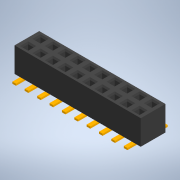
# Autodesk Inventor part: SMT10x2pin
Saved by Autodesk Inventor 2022 (Build 260153000, 153)
## iProperties
Created: 2024-12-15
Part Number: SMT10x2pin
Material: Типовые
Document SubType Name: Modeling
Designer: Andrey
Density: 1 g/cm^3
Appearance: По умолчанию
Author: Andrey
Autodesk Inventor part; units mm, degrees
ref_plane "YZ Plane" through (0, 0, 0) normal (1, 0, 0) x (0, 1, 0)
ref_plane "XZ Plane" through (0, 0, 0) normal (0, 1, 0) x (-1, 0, 0)
ref_plane "XY Plane" through (0, 0, 0) normal (0, 0, 1) x (1, 0, 0)
sketch "Эскиз1" plane through (0, 0, 0) normal (0, 1, 0) x (-1, 0, 0)
  line L0 (-10.2, 2) -> (10.2, 2)
  line L1 (10.2, 2) -> (10.2, -2)
  line L2 (10.2, -2) -> (-10.2, -2)
  line L3 (-10.2, -2) -> (-10.2, 2)
  line L4 (-10.2, 2) -> (10.2, -2) construction
  line L5 (10.2, 2) -> (-10.2, -2) construction
  line L6 (-9, 1) -> (9, 1)
  line L7 (9, 1) -> (9, -1)
  line L8 (9, -1) -> (-9, -1)
  line L9 (-9, -1) -> (-9, 1)
  line L10 (-9, 1) -> (9, -1) construction
  line L11 (9, 1) -> (-9, -1) construction
  line L12 (9.45, 1.45) -> (8.55, 1.45)
  line L13 (8.55, 1.45) -> (8.55, 0.55)
  line L14 (8.55, 0.55) -> (9.45, 0.55)
  line L15 (9.45, 0.55) -> (9.45, 1.45)
  line L16 (9.45, 1.45) -> (8.55, 0.55) construction
  line L17 (8.55, 1.45) -> (9.45, 0.55) construction
  line L18 (9, 1) -> (7, 1)
  line L19 (7, 1) -> (5, 1)
  line L20 (5, 1) -> (3, 1)
  line L21 (3, 1) -> (1, 1)
  line L22 (1, 1) -> (-1, 1)
  line L23 (-1, 1) -> (-3, 1)
  line L24 (-3, 1) -> (-5, 1)
  line L25 (-5, 1) -> (-7, 1)
  line L26 (9, -1) -> (7, -1)
  line L27 (7, -1) -> (5, -1)
  line L28 (5, -1) -> (3, -1)
  line L29 (3, -1) -> (1, -1)
  line L30 (1, -1) -> (-1, -1)
  line L31 (-1, -1) -> (-3, -1)
  line L32 (-3, -1) -> (-5, -1)
  line L33 (-5, -1) -> (-7, -1)
  line L34 (7.45, 1.45) -> (6.55, 1.45)
  line L35 (6.55, 1.45) -> (6.55, 0.55)
  line L36 (6.55, 0.55) -> (7.45, 0.55)
  line L37 (7.45, 0.55) -> (7.45, 1.45)
  line L38 (7.45, 1.45) -> (6.55, 0.55) construction
  line L39 (6.55, 1.45) -> (7.45, 0.55) construction
  line L40 (5.45, 1.45) -> (4.55, 1.45)
  line L41 (4.55, 1.45) -> (4.55, 0.55)
  line L42 (4.55, 0.55) -> (5.45, 0.55)
  line L43 (5.45, 0.55) -> (5.45, 1.45)
  line L44 (5.45, 1.45) -> (4.55, 0.55) construction
  line L45 (4.55, 1.45) -> (5.45, 0.55) construction
  line L46 (3.45, 1.45) -> (2.55, 1.45)
  line L47 (2.55, 1.45) -> (2.55, 0.55)
  line L48 (2.55, 0.55) -> (3.45, 0.55)
  line L49 (3.45, 0.55) -> (3.45, 1.45)
  line L50 (3.45, 1.45) -> (2.55, 0.55) construction
  line L51 (2.55, 1.45) -> (3.45, 0.55) construction
  line L52 (1.45, 1.45) -> (0.55, 1.45)
  line L53 (0.55, 1.45) -> (0.55, 0.55)
  line L54 (0.55, 0.55) -> (1.45, 0.55)
  line L55 (1.45, 0.55) -> (1.45, 1.45)
  line L56 (1.45, 1.45) -> (0.55, 0.55) construction
  line L57 (0.55, 1.45) -> (1.45, 0.55) construction
  line L58 (-0.55, 1.45) -> (-1.45, 1.45)
  line L59 (-1.45, 1.45) -> (-1.45, 0.55)
  line L60 (-1.45, 0.55) -> (-0.55, 0.55)
  line L61 (-0.55, 0.55) -> (-0.55, 1.45)
  line L62 (-0.55, 1.45) -> (-1.45, 0.55) construction
  line L63 (-1.45, 1.45) -> (-0.55, 0.55) construction
  line L64 (-2.55, 1.45) -> (-3.45, 1.45)
  line L65 (-3.45, 1.45) -> (-3.45, 0.55)
  line L66 (-3.45, 0.55) -> (-2.55, 0.55)
  line L67 (-2.55, 0.55) -> (-2.55, 1.45)
  line L68 (-2.55, 1.45) -> (-3.45, 0.55) construction
  line L69 (-3.45, 1.45) -> (-2.55, 0.55) construction
  line L70 (-4.55, 1.45) -> (-5.45, 1.45)
  line L71 (-5.45, 1.45) -> (-5.45, 0.55)
  line L72 (-5.45, 0.55) -> (-4.55, 0.55)
  line L73 (-4.55, 0.55) -> (-4.55, 1.45)
  line L74 (-4.55, 1.45) -> (-5.45, 0.55) construction
  line L75 (-5.45, 1.45) -> (-4.55, 0.55) construction
  line L76 (-6.55, 1.45) -> (-7.45, 1.45)
  line L77 (-7.45, 1.45) -> (-7.45, 0.55)
  line L78 (-7.45, 0.55) -> (-6.55, 0.55)
  line L79 (-6.55, 0.55) -> (-6.55, 1.45)
  line L80 (-6.55, 1.45) -> (-7.45, 0.55) construction
  line L81 (-7.45, 1.45) -> (-6.55, 0.55) construction
  line L82 (-8.55, 1.45) -> (-9.45, 1.45)
  line L83 (-9.45, 1.45) -> (-9.45, 0.55)
  line L84 (-9.45, 0.55) -> (-8.55, 0.55)
  line L85 (-8.55, 0.55) -> (-8.55, 1.45)
  line L86 (-8.55, 1.45) -> (-9.45, 0.55) construction
  line L87 (-9.45, 1.45) -> (-8.55, 0.55) construction
  line L88 (-8.55, -0.55) -> (-9.45, -0.55)
  line L89 (-9.45, -0.55) -> (-9.45, -1.45)
  line L90 (-9.45, -1.45) -> (-8.55, -1.45)
  line L91 (-8.55, -1.45) -> (-8.55, -0.55)
  line L92 (-8.55, -0.55) -> (-9.45, -1.45) construction
  line L93 (-9.45, -0.55) -> (-8.55, -1.45) construction
  line L94 (-6.55, -0.55) -> (-7.45, -0.55)
  line L95 (-7.45, -0.55) -> (-7.45, -1.45)
  line L96 (-7.45, -1.45) -> (-6.55, -1.45)
  line L97 (-6.55, -1.45) -> (-6.55, -0.55)
  line L98 (-6.55, -0.55) -> (-7.45, -1.45) construction
  line L99 (-7.45, -0.55) -> (-6.55, -1.45) construction
  line L100 (-4.55, -0.55) -> (-5.45, -0.55)
  line L101 (-5.45, -0.55) -> (-5.45, -1.45)
  line L102 (-5.45, -1.45) -> (-4.55, -1.45)
  line L103 (-4.55, -1.45) -> (-4.55, -0.55)
  line L104 (-4.55, -0.55) -> (-5.45, -1.45) construction
  line L105 (-5.45, -0.55) -> (-4.55, -1.45) construction
  line L106 (-0.5574, -0.5122) -> (-1.4574, -0.5122)
  line L107 (-1.4574, -0.5122) -> (-1.4574, -1.4122)
  line L108 (-1.4574, -1.4122) -> (-0.5574, -1.4122)
  line L109 (-0.5574, -1.4122) -> (-0.5574, -0.5122)
  line L110 (-0.5574, -0.5122) -> (-1.4574, -1.4122) construction
  line L111 (-1.4574, -0.5122) -> (-0.5574, -1.4122) construction
  line L112 (-2.55, -0.55) -> (-3.45, -0.55)
  line L113 (-3.45, -0.55) -> (-3.45, -1.45)
  line L114 (-3.45, -1.45) -> (-2.55, -1.45)
  line L115 (-2.55, -1.45) -> (-2.55, -0.55)
  line L116 (-2.55, -0.55) -> (-3.45, -1.45) construction
  line L117 (-3.45, -0.55) -> (-2.55, -1.45) construction
  line L118 (9.45, -0.55) -> (8.55, -0.55)
  line L119 (8.55, -0.55) -> (8.55, -1.45)
  line L120 (8.55, -1.45) -> (9.45, -1.45)
  line L121 (9.45, -1.45) -> (9.45, -0.55)
  line L122 (9.45, -0.55) -> (8.55, -1.45) construction
  line L123 (8.55, -0.55) -> (9.45, -1.45) construction
  line L124 (9, -1) -> (7, -1)
  line L125 (7, -1) -> (5, -1)
  line L126 (5, -1) -> (3, -1)
  line L127 (3, -1) -> (1, -1)
  line L128 (7.45, -0.55) -> (6.55, -0.55)
  line L129 (6.55, -0.55) -> (6.55, -1.45)
  line L130 (6.55, -1.45) -> (7.45, -1.45)
  line L131 (7.45, -1.45) -> (7.45, -0.55)
  line L132 (7.45, -0.55) -> (6.55, -1.45) construction
  line L133 (6.55, -0.55) -> (7.45, -1.45) construction
  line L134 (5.45, -0.55) -> (4.55, -0.55)
  line L135 (4.55, -0.55) -> (4.55, -1.45)
  line L136 (4.55, -1.45) -> (5.45, -1.45)
  line L137 (5.45, -1.45) -> (5.45, -0.55)
  line L138 (5.45, -0.55) -> (4.55, -1.45) construction
  line L139 (4.55, -0.55) -> (5.45, -1.45) construction
  line L140 (3.45, -0.55) -> (2.55, -0.55)
  line L141 (2.55, -0.55) -> (2.55, -1.45)
  line L142 (2.55, -1.45) -> (3.45, -1.45)
  line L143 (3.45, -1.45) -> (3.45, -0.55)
  line L144 (3.45, -0.55) -> (2.55, -1.45) construction
  line L145 (2.55, -0.55) -> (3.45, -1.45) construction
  line L146 (1.45, -0.55) -> (0.55, -0.55)
  line L147 (0.55, -0.55) -> (0.55, -1.45)
  line L148 (0.55, -1.45) -> (1.45, -1.45)
  line L149 (1.45, -1.45) -> (1.45, -0.55)
  line L150 (1.45, -0.55) -> (0.55, -1.45) construction
  line L151 (0.55, -0.55) -> (1.45, -1.45) construction
  point P0 (0, 0)
  point P1 (3, 1)
  point P2 (-1, 1)
  point P3 (-5, 1)
  point P4 (-7, 1)
  point P5 (-7, -1)
  point P6 (-5, -1)
  point P7 (-1.0074, -0.9622)
  point P8 (-3, -1)
  point P9 (3, -1)
  dimension "d0" = 20.4
  dimension "d1" = 4
  dimension "d2" = 18
  dimension "d3" = 2
  dimension "d4" = 0.9
  dimension "d5" = 0.9
  dimension "d6" = 2
  dimension "d7" = 2
  dimension "d8" = 2
  dimension "d9" = 2
  dimension "d10" = 2
  dimension "d11" = 2
  dimension "d12" = 2
  dimension "d13" = 2
  dimension "d14" = 2
  dimension "d15" = 2
  dimension "d16" = 2
  dimension "d17" = 2
  dimension "d18" = 2
  dimension "d19" = 2
  dimension "d20" = 2
  dimension "d21" = 2
  dimension "d22" = 0.9
  dimension "d23" = 0.9
  dimension "d24" = 0.9
  dimension "d25" = 0.9
  dimension "d26" = 0.9
  dimension "d27" = 0.9
  dimension "d28" = 0.9
  dimension "d29" = 0.9
  dimension "d30" = 0.9
  dimension "d31" = 0.9
  dimension "d32" = 0.9
  dimension "d33" = 0.9
  dimension "d34" = 0.9
  dimension "d35" = 0.9
  dimension "d36" = 0.9
  dimension "d37" = 0.9
  dimension "d38" = 0.9
  dimension "d39" = 0.9
  dimension "d40" = 0.9
  dimension "d41" = 0.9
  dimension "d42" = 0.9
  dimension "d43" = 0.9
  dimension "d44" = 0.9
  dimension "d45" = 0.9
  dimension "d46" = 0.9
  dimension "d47" = 0.9
  dimension "d48" = 0.9
  dimension "d49" = 0.9
  dimension "d50" = 0.9
  dimension "d51" = 0.9
  dimension "d52" = 2
  dimension "d53" = 2
  dimension "d54" = 2
  dimension "d55" = 2
  dimension "d56" = 0.9
  dimension "d57" = 0.9
  dimension "d58" = 0.9
  dimension "d59" = 0.9
  dimension "d60" = 0.9
  dimension "d61" = 0.9
  dimension "d62" = 0.9
  dimension "d63" = 0.9
  constraints: 300 end point, 44 midpoint, 43 parallel, 21 horizontal, 21 perpendicular, 1 vertical, 22 other
  measures "d0" distance of L1.end L2.end
  measures "d1" distance of L0.end L1.end
  measures "d2" distance of L7.end L9.start
  measures "d3" distance of L7.start L7.end
  measures "d4" distance of L14.end L13.end
  measures "d5" distance of L13.end L12.end
  measures "d6" distance of L7.start L18.end
  measures "d7" distance of L18.end L19.end
  measures "d8" distance of L19.end L20.end
  measures "d9" distance of L20.end L21.end
  measures "d10" distance of L21.end L22.end
  measures "d11" distance of L22.end L23.end
  measures "d12" distance of L23.end L24.end
  measures "d13" distance of L24.end L25.end
  measures "d14" distance of L7.end L26.end
  measures "d15" distance of L26.end L27.end
  measures "d16" distance of L27.end L28.end
  measures "d17" distance of L28.end L29.end
  measures "d18" distance of L29.end L30.end
  measures "d19" distance of L30.end L31.end
  measures "d20" distance of L31.end L32.end
  measures "d21" distance of L32.end L33.end
  measures "d22" distance of L36.end L35.end
  measures "d23" distance of L35.end L34.end
  measures "d24" distance of L42.end L41.end
  measures "d25" distance of L41.end L40.end
  measures "d26" distance of L48.end L47.end
  measures "d27" distance of L47.end L46.end
  measures "d28" distance of L54.end L53.end
  measures "d29" distance of L53.end L52.end
  measures "d30" distance of L60.end L59.end
  measures "d31" distance of L59.end L58.end
  measures "d32" distance of L66.end L65.end
  measures "d33" distance of L65.end L64.end
  measures "d34" distance of L72.end L71.end
  measures "d35" distance of L71.end L70.end
  measures "d36" distance of L78.end L77.end
  measures "d37" distance of L77.end L76.end
  measures "d38" distance of L84.end L83.end
  measures "d39" distance of L83.end L82.end
  measures "d40" distance of L90.end L89.end
  measures "d41" distance of L89.end L88.end
  measures "d42" distance of L96.end L95.end
  measures "d43" distance of L95.end L94.end
  measures "d44" distance of L102.end L101.end
  measures "d45" distance of L101.end L100.end
  measures "d46" distance of L108.end L107.end
  measures "d47" distance of L107.end L106.end
  measures "d48" distance of L114.end L113.end
  measures "d49" distance of L113.end L112.end
  measures "d50" distance of L121.start L119.end
  measures "d51" distance of L119.end L118.end
  measures "d52" distance of L124.start L125.start
  measures "d53" distance of L125.start L125.end
  measures "d54" distance of L125.end L126.end
  measures "d55" distance of L126.end L127.end
  measures "d56" distance of L130.end L129.end
  measures "d57" distance of L129.end L129.start
  measures "d58" distance of L137.start L135.end
  measures "d59" distance of L135.end L135.start
  measures "d60" distance of L142.end L141.end
  measures "d61" distance of L141.end L141.start
  measures "d62" distance of L149.start L148.start
  measures "d63" distance of L148.start L147.start
extrude "Выдавливание1" add sketch "Эскиз1" along normal blind 4 contours L0 L1 L2 L3 | L6 L77 L78 L79 L71 L72 L73 L65 L66 L67 L59 L60 L61 L53 L54 L55 L47 L48 L49 L41 L42 L43 L35 L36 L37 L13 L14 L7 L118 L119 L8 L131 L128 L129 L137 L134 L135 L143 L140 L141 L149 L146 L147 L109 L106 L107 L115 L112 L113 L103 L100 L101 L97 L94 L95 L91 L88 L9 L84 L85
chamfer "Фаска1" distance 0.2 angle 45 80 edges at (4.55, 4, 1) (5.45, 4, 1) (5, 4, -0.55) (-8.55, 4, 1) (-9, 4, 1.45) (-9.45, 4, 1) (-9.45, 4, -1) (-9, 4, 0.55) (-9, 4, -0.55) (-1.45, 4, 1) (-2.55, 4, 1) (3.45, 4, -1) (2.55, 4, -1) (-3.45, 4, -1) (-2.55, 4, -1) (-3, 4, -0.55) (-3, 4, -1.45) (-3, 4, 1.45) (-3, 4, 0.55) (-3.45, 4, 1) (-4.55, 4, 1) (-5, 4, 1.45) (-7.45, 4, -1) (-7, 4, -1.45) (-6.55, 4, -1) (-7, 4, -0.55) (-5, 4, 0.55) (-6.55, 4, 1) (-7.45, 4, 1) (-7, 4, 0.55) (-5.45, 4, 1) (-7, 4, 1.45) (-8.55, 4, -1) (-9, 4, -1.45) (-5.45, 4, -1) (-5, 4, -1.45) (-4.55, 4, -1) (-5, 4, -0.55) (-1.45, 4, -1) (-0.55, 4, -1) (-1, 4, -1.45) (-1, 4, -0.55) (-1, 4, 0.55) (0.55, 4, 1) (-0.55, 4, 1) (1.45, 4, 1) (1, 4, 0.55) (1, 4, 1.45) (1.4574, 4, -0.9622) (0.5574, 4, -0.9622) (1.0074, 4, -1.4122) (1.0074, 4, -0.5122) (-1, 4, 1.45) (2.55, 4, 1) (3, 4, -0.55) (3, 4, 0.55) (3, 4, 1.45) (3.45, 4, 1) (5, 4, 0.55) (5, 4, 1.45) (5.45, 4, -1) (4.55, 4, -1) (5, 4, -1.45) (6.55, 4, -1) (7, 4, -1.45) (7.45, 4, -1) (7, 4, -0.55) (7.45, 4, 1) (7, 4, 1.45) (6.55, 4, 1) (7, 4, 0.55) (8.55, 4, -1) (9, 4, -1.45) (9.45, 4, -1) (9, 4, -0.55) (9, 4, 0.55) (9.45, 4, 1) (9, 4, 1.45) (8.55, 4, 1) (3, 4, -1.45)
sketch "Эскиз2" plane through (0, 0, 0) normal (0, -1, 0) x (1, 0, 0)
  line L0 (-9.45, 0.55) -> (-8.55, 0.55) projected
  line L1 (-9, 0.55) -> (-9, -0.55)
  line L2 (-8.55, -0.55) -> (-9.45, -0.55) projected
  line L3 (10.2, -2) -> (-10.2, -2) projected
  line L4 (10.2, 2) -> (10.2, -2) projected
  line L5 (-10.2, 2) -> (10.2, 2) projected
  line L6 (-10.2, -2) -> (-10.2, 2) projected
  line L7 (-8.55, 0.55) -> (-8.55, 1.45) projected
  line L8 (-9.45, 0.55) -> (-8.55, 0.55) projected
  line L9 (-9.45, 1.45) -> (-9.45, 0.55) projected
  line L10 (-8.55, 1.45) -> (-9.45, 1.45) projected
  line L11 (-8.55, -0.55) -> (-9.45, -0.55) projected
  line L12 (-8.55, -1.45) -> (-8.55, -0.55) projected
  line L13 (-9.45, -1.45) -> (-8.55, -1.45) projected
  line L14 (-9.45, -0.55) -> (-9.45, -1.45) projected
  line L15 (-7.45, -0.55) -> (-7.45, -1.45) projected
  line L16 (-6.55, -0.55) -> (-7.45, -0.55) projected
  line L17 (-6.55, -1.45) -> (-6.55, -0.55) projected
  line L18 (-7.45, -1.45) -> (-6.55, -1.45) projected
  line L19 (-5.45, -0.55) -> (-5.45, -1.45) projected
  line L20 (-4.55, -0.55) -> (-5.45, -0.55) projected
  line L21 (-4.55, -1.45) -> (-4.55, -0.55) projected
  line L22 (-5.45, -1.45) -> (-4.55, -1.45) projected
  line L23 (-3.45, -0.55) -> (-3.45, -1.45) projected
  line L24 (-2.55, -0.55) -> (-3.45, -0.55) projected
  line L25 (-2.55, -1.45) -> (-2.55, -0.55) projected
  line L26 (-3.45, -1.45) -> (-2.55, -1.45) projected
  line L27 (-1.45, -0.55) -> (-1.45, -1.45) projected
  line L28 (-0.55, -0.55) -> (-1.45, -0.55) projected
  line L29 (-0.55, -1.45) -> (-0.55, -0.55) projected
  line L30 (-1.45, -1.45) -> (-0.55, -1.45) projected
  line L31 (0.5574, -0.5122) -> (0.5574, -1.4122) projected
  line L32 (1.4574, -0.5122) -> (0.5574, -0.5122) projected
  line L33 (1.4574, -1.4122) -> (1.4574, -0.5122) projected
  line L34 (0.5574, -1.4122) -> (1.4574, -1.4122) projected
  line L35 (2.55, -0.55) -> (2.55, -1.45) projected
  line L36 (3.45, -0.55) -> (2.55, -0.55) projected
  line L37 (3.45, -1.45) -> (3.45, -0.55) projected
  line L38 (2.55, -1.45) -> (3.45, -1.45) projected
  line L39 (4.55, -0.55) -> (4.55, -1.45) projected
  line L40 (5.45, -0.55) -> (4.55, -0.55) projected
  line L41 (5.45, -1.45) -> (5.45, -0.55) projected
  line L42 (4.55, -1.45) -> (5.45, -1.45) projected
  line L43 (6.55, -0.55) -> (6.55, -1.45) projected
  line L44 (7.45, -0.55) -> (6.55, -0.55) projected
  line L45 (7.45, -1.45) -> (7.45, -0.55) projected
  line L46 (6.55, -1.45) -> (7.45, -1.45) projected
  line L47 (8.55, -0.55) -> (8.55, -1.45) projected
  line L48 (9.45, -0.55) -> (8.55, -0.55) projected
  line L49 (9.45, -1.45) -> (9.45, -0.55) projected
  line L50 (8.55, -1.45) -> (9.45, -1.45) projected
  line L51 (8.55, 0.55) -> (9.45, 0.55) projected
  line L52 (8.55, 1.45) -> (8.55, 0.55) projected
  line L53 (9.45, 1.45) -> (8.55, 1.45) projected
  line L54 (9.45, 0.55) -> (9.45, 1.45) projected
  line L55 (7.45, 0.55) -> (7.45, 1.45) projected
  line L56 (6.55, 0.55) -> (7.45, 0.55) projected
  line L57 (6.55, 1.45) -> (6.55, 0.55) projected
  line L58 (7.45, 1.45) -> (6.55, 1.45) projected
  line L59 (5.45, 0.55) -> (5.45, 1.45) projected
  line L60 (4.55, 0.55) -> (5.45, 0.55) projected
  line L61 (4.55, 1.45) -> (4.55, 0.55) projected
  line L62 (5.45, 1.45) -> (4.55, 1.45) projected
  line L63 (3.45, 0.55) -> (3.45, 1.45) projected
  line L64 (2.55, 0.55) -> (3.45, 0.55) projected
  line L65 (2.55, 1.45) -> (2.55, 0.55) projected
  line L66 (3.45, 1.45) -> (2.55, 1.45) projected
  line L67 (1.45, 0.55) -> (1.45, 1.45) projected
  line L68 (0.55, 0.55) -> (1.45, 0.55) projected
  line L69 (0.55, 1.45) -> (0.55, 0.55) projected
  line L70 (1.45, 1.45) -> (0.55, 1.45) projected
  line L71 (-0.55, 0.55) -> (-0.55, 1.45) projected
  line L72 (-1.45, 0.55) -> (-0.55, 0.55) projected
  line L73 (-1.45, 1.45) -> (-1.45, 0.55) projected
  line L74 (-0.55, 1.45) -> (-1.45, 1.45) projected
  line L75 (-2.55, 0.55) -> (-2.55, 1.45) projected
  line L76 (-3.45, 0.55) -> (-2.55, 0.55) projected
  line L77 (-3.45, 1.45) -> (-3.45, 0.55) projected
  line L78 (-2.55, 1.45) -> (-3.45, 1.45) projected
  line L79 (-4.55, 0.55) -> (-4.55, 1.45) projected
  line L80 (-5.45, 0.55) -> (-4.55, 0.55) projected
  line L81 (-5.45, 1.45) -> (-5.45, 0.55) projected
  line L82 (-4.55, 1.45) -> (-5.45, 1.45) projected
  line L83 (-7.45, 1.45) -> (-7.45, 0.55) projected
  line L84 (-6.55, 1.45) -> (-7.45, 1.45) projected
  line L85 (-6.55, 0.55) -> (-6.55, 1.45) projected
  line L86 (-7.45, 0.55) -> (-6.55, 0.55) projected
  line L87 (-9.3, -3.25) -> (-8.7, -3.25)
  line L88 (-8.7, -3.25) -> (-8.7, 3.25)
  line L89 (-8.7, 3.25) -> (-9.3, 3.25)
  line L90 (-9.3, 3.25) -> (-9.3, -3.25)
  line L91 (-9.3, -3.25) -> (-8.7, 3.25) construction
  line L92 (-8.7, -3.25) -> (-9.3, 3.25) construction
  line L93 (-7, 0.55) -> (-7, -0.55)
  line L94 (-7.3, -3.25) -> (-6.7, -3.25)
  line L95 (-6.7, -3.25) -> (-6.7, 3.25)
  line L96 (-6.7, 3.25) -> (-7.3, 3.25)
  line L97 (-7.3, 3.25) -> (-7.3, -3.25)
  line L98 (-7.3, -3.25) -> (-6.7, 3.25) construction
  line L99 (-6.7, -3.25) -> (-7.3, 3.25) construction
  line L100 (-5, 0.55) -> (-5, -0.55)
  line L101 (-5.3, -3.25) -> (-4.7, -3.25)
  line L102 (-4.7, -3.25) -> (-4.7, 3.25)
  line L103 (-4.7, 3.25) -> (-5.3, 3.25)
  line L104 (-5.3, 3.25) -> (-5.3, -3.25)
  line L105 (-5.3, -3.25) -> (-4.7, 3.25) construction
  line L106 (-4.7, -3.25) -> (-5.3, 3.25) construction
  line L107 (-3, 0.55) -> (-3, -0.55)
  line L108 (-3.3, -3.25) -> (-2.7, -3.25)
  line L109 (-2.7, -3.25) -> (-2.7, 3.25)
  line L110 (-2.7, 3.25) -> (-3.3, 3.25)
  line L111 (-3.3, 3.25) -> (-3.3, -3.25)
  line L112 (-3.3, -3.25) -> (-2.7, 3.25) construction
  line L113 (-2.7, -3.25) -> (-3.3, 3.25) construction
  line L114 (-1, 0.55) -> (-1, -0.55)
  line L115 (-1.3, -3.25) -> (-0.7, -3.25)
  line L116 (-0.7, -3.25) -> (-0.7, 3.25)
  line L117 (-0.7, 3.25) -> (-1.3, 3.25)
  line L118 (-1.3, 3.25) -> (-1.3, -3.25)
  line L119 (-1.3, -3.25) -> (-0.7, 3.25) construction
  line L120 (-0.7, -3.25) -> (-1.3, 3.25) construction
  line L121 (1, 0.55) -> (1, -0.55)
  line L122 (0.7, -3.25) -> (1.3, -3.25)
  line L123 (1.3, -3.25) -> (1.3, 3.25)
  line L124 (1.3, 3.25) -> (0.7, 3.25)
  line L125 (0.7, 3.25) -> (0.7, -3.25)
  line L126 (0.7, -3.25) -> (1.3, 3.25) construction
  line L127 (1.3, -3.25) -> (0.7, 3.25) construction
  line L128 (3, 0.55) -> (3, -0.55)
  line L129 (2.7, -3.25) -> (3.3, -3.25)
  line L130 (3.3, -3.25) -> (3.3, 3.25)
  line L131 (3.3, 3.25) -> (2.7, 3.25)
  line L132 (2.7, 3.25) -> (2.7, -3.25)
  line L133 (2.7, -3.25) -> (3.3, 3.25) construction
  line L134 (3.3, -3.25) -> (2.7, 3.25) construction
  line L135 (5, 0.55) -> (5, -0.55)
  line L136 (4.7, -3.25) -> (5.3, -3.25)
  line L137 (5.3, -3.25) -> (5.3, 3.25)
  line L138 (5.3, 3.25) -> (4.7, 3.25)
  line L139 (4.7, 3.25) -> (4.7, -3.25)
  line L140 (4.7, -3.25) -> (5.3, 3.25) construction
  line L141 (5.3, -3.25) -> (4.7, 3.25) construction
  line L142 (7, 0.55) -> (7, -0.55)
  line L143 (6.7, -3.25) -> (7.3, -3.25)
  line L144 (7.3, -3.25) -> (7.3, 3.25)
  line L145 (7.3, 3.25) -> (6.7, 3.25)
  line L146 (6.7, 3.25) -> (6.7, -3.25)
  line L147 (6.7, -3.25) -> (7.3, 3.25) construction
  line L148 (7.3, -3.25) -> (6.7, 3.25) construction
  line L149 (9, 0.55) -> (9, -0.55)
  line L150 (8.7, -3.25) -> (9.3, -3.25)
  line L151 (9.3, -3.25) -> (9.3, 3.25)
  line L152 (9.3, 3.25) -> (8.7, 3.25)
  line L153 (8.7, 3.25) -> (8.7, -3.25)
  line L154 (8.7, -3.25) -> (9.3, 3.25) construction
  line L155 (9.3, -3.25) -> (8.7, 3.25) construction
  point P0 (0, 0)
  point P1 (-9, 0)
  point P2 (-9.3, -1.45)
  point P3 (-8.7, -1.45)
  point P4 (-9.3, 1.45)
  point P5 (-8.7, 1.45)
  point P6 (-7, 0)
  point P7 (-5, 0)
  point P8 (-3, 0)
  point P9 (-1, 0)
  point P10 (1, 0)
  point P11 (3, 0)
  point P12 (5, 0)
  point P13 (7, 0)
  point P14 (9, 0)
  point P15 (6.7, 1.45)
  point P16 (7.3, 1.45)
  point P17 (8.7, 1.45)
  point P18 (9.3, 1.45)
  point P19 (4.7, 1.45)
  point P20 (5.3, 1.45)
  point P21 (2.7, 1.45)
  point P22 (3.3, 1.45)
  point P23 (0.7, 1.45)
  point P24 (1.3, 1.45)
  point P25 (-1.3, 1.45)
  point P26 (-0.7, 1.45)
  point P27 (-3.3, 1.45)
  point P28 (-2.7, 1.45)
  point P29 (7.3, -1.45)
  point P30 (6.7, -1.45)
  point P31 (9.3, -1.45)
  point P32 (8.7, -1.45)
  point P33 (5.3, -1.45)
  point P34 (4.7, -1.45)
  point P35 (3.3, -1.45)
  point P36 (2.7, -1.45)
  point P37 (1.3, -1.4122)
  point P38 (0.7, -1.4122)
  point P39 (-0.7, -1.45)
  point P40 (-1.3, -1.45)
  point P41 (-2.7, -1.45)
  point P42 (-3.3, -1.45)
  point P43 (-5.3, -1.45)
  point P44 (-4.7, -1.45)
  point P45 (-5.3, 1.45)
  point P46 (-4.7, 1.45)
  point P47 (-7.3, 1.45)
  point P48 (-6.7, 1.45)
  point P49 (-6.7, -1.45)
  point P50 (-7.3, -1.45)
  dimension "d69" = 0.6
  dimension "d70" = 6.5
  dimension "d91" = 0.6
  dimension "d92" = 6.5
  dimension "d93" = 0.6
  dimension "d94" = 6.5
  dimension "d95" = 0.6
  dimension "d96" = 6.5
  dimension "d97" = 0.6
  dimension "d98" = 6.5
  dimension "d99" = 0.6
  dimension "d100" = 6.5
  dimension "d101" = 0.6
  dimension "d102" = 6.5
  dimension "d103" = 0.6
  dimension "d104" = 6.5
  dimension "d105" = 0.6
  dimension "d106" = 6.5
  dimension "d107" = 0.6
  dimension "d108" = 6.5
  constraints: 140 end point, 32 midpoint, 20 parallel, 10 horizontal, 10 perpendicular
  measures "d69" distance between parallel lines of L88 L90
  measures "d70" distance of L89.end L87.start
  measures "d91" distance between parallel lines of L95 L97
  measures "d92" distance of L99.end L94.start
  measures "d93" distance between parallel lines of L102 L104
  measures "d94" distance of L106.end L101.start
  measures "d95" distance between parallel lines of L109 L111
  measures "d96" distance of L113.end L108.start
  measures "d97" distance between parallel lines of L116 L118
  measures "d98" distance of L120.end L115.start
  measures "d99" distance between parallel lines of L123 L125
  measures "d100" distance of L127.end L122.start
  measures "d101" distance between parallel lines of L130 L132
  measures "d102" distance of L134.end L129.start
  measures "d103" distance between parallel lines of L137 L139
  measures "d104" distance of L141.end L136.start
  measures "d105" distance between parallel lines of L144 L146
  measures "d106" distance of L148.end L143.start
  measures "d107" distance between parallel lines of L151 L153
  measures "d108" distance of L155.end L150.start
extrude "Выдавливание2" add sketch "Эскиз2" along normal blind 0.3 contours L90 L5 L88 L10 | L90 L89 L88 L5 | L13 L88 L3 L90 | L3 L88 L87 L90 | L97 L96 L95 L5 | L5 L95 L84 L97 | L97 L18 L95 L3 | L3 L95 L94 L97 | L104 L103 L102 L5 | L5 L102 L82 L104 | L104 L22 L102 L3 | L3 L102 L101 L104 | L111 L110 L109 L5 | L5 L109 L78 L111 | L111 L26 L109 L3 | L3 L109 L108 L111 | L118 L117 L116 L5 | L5 L116 L74 L118 | L118 L30 L116 L3 | L3 L116 L115 L118 | L125 L124 L123 L5 | L5 L123 L70 L125 | L125 L34 L123 L3 | L3 L123 L122 L125 | L132 L131 L130 L5 | L5 L130 L66 L132 | L132 L38 L130 L3 | L3 L130 L129 L132 | L139 L138 L137 L5 | L5 L137 L62 L139 | L139 L42 L137 L3 | L3 L137 L136 L139 | L146 L145 L144 L5 | L5 L144 L58 L146 | L146 L46 L144 L3 | L3 L144 L143 L146 | L153 L152 L151 L5 | L5 L151 L53 L153 | L153 L50 L151 L3 | L3 L151 L150 L153
